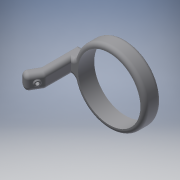
# Autodesk Inventor part: Layer1Gear
Saved by Autodesk Inventor 2019 (Build 230136000, 136)
## iProperties
Created: 2022-08-24
Part Number: Layer1Gear
Material: Generic
Document SubType Name: Modeling
Designer: zreik
Density: 1 g/cm^3
Appearance: Default
Author: zreik
Autodesk Inventor part; units mm, degrees
note: some values were not read from the file. Chosen so that the rebuilt part matches the saved one: sketch regions of "Extrusion1"; arc direction of "Extrusion1".
ref_plane "YZ Plane" through (0, 0, 0) normal (1, 0, 0) x (0, 1, 0)
ref_plane "XZ Plane" through (0, 0, 0) normal (0, 1, 0) x (-1, 0, 0)
ref_plane "XY Plane" through (0, 0, 0) normal (0, 0, 1) x (1, 0, 0)
sketch "Sketch1" plane through (0, 0, 0) normal (0, 0, 1) x (1, 0, 0)
  circle A0 centre (0, 0) radius 32.75
  circle A1 centre (0, 0) radius 37.75
  line L0 (-31.879657, 7.5) -> (-40, 7.5)
  line L1 (-40, 7.5) -> (-40, -7.5)
  line L2 (-40, -7.5) -> (-31.879657, -7.5)
  dimension "d0" = 65.5
  dimension "d1" = 75.5
  dimension "d4" = 15
  dimension "d5" = 40
  dimension "d6" = 7.5
  constraints: 6 end point, 2 centre point, 2 coincident, 2 perpendicular, 2 point on circle, 1 horizontal
  measures "d0" diameter of A0
  measures "d1" diameter of A1
  measures "d4" distance between parallel lines of L0 L2
  measures "d5" distance from line of point (0, 0) L1
  measures "d6" distance from line of point (0, 0) L0
extrude "Extrusion1" add sketch "Sketch1" along normal blind 17 contours A0 L0 A1 L2 | A0 L2 A1 L0 | A1 L2 L1 L0
chamfer "Chamfer1" distance 2 angle 45 2 edges at (-36.9975, 7.5, 8.5) (-36.9975, -7.5, 8.5)
fillet "Fillet1" radius 2 4 edges at (-38.9975, 7.5, 8.5) (-36.5483, 9.4489, 8.5) (-36.5483, -9.4489, 8.5) (-38.9975, -7.5, 8.5)
sketch "Sketch2" plane through (0, 0, 0) normal (0, 0, -1) x (-1, 0, 0)
  line L0 (40, 7.5) -> (40, -7.5)
  line L1 (40, -7.5) -> (50, -7.5)
  line L2 (50, -7.5) -> (50, 7.5)
  line L3 (50, 7.5) -> (40, 7.5)
  line L4 (40, 7.5) -> (40, -7.5)
  line L5 (39.696118, 7.5) -> (40, 7.5)
  point P0 (0, 0)
  point P1 (36.401408, 10)
  dimension "d11" = 10
  dimension "d12" = 0
  constraints: 8 end point, 2 parallel, 1 horizontal, 1 perpendicular, 1 other
  measures "d11" distance of L2.end L3.end
  measures "d12" vertical extent of L3
extrude "Extrusion2" add sketch "Sketch2" against normal blind 59
chamfer_without_effect "Chamfer2"
sketch "Sketch4" plane through (-41.339746, -7.5, 59) normal (-0.5, 0, 0.8660254) x (0.8660254, 0, 0.5)
  line L0 (0, 0) -> (-10, 0)
  line L1 (-10, 15) -> (0, 15)
  line L2 (-19.839746, 0) -> (1.160254, 0)
  line L3 (-37, 15) -> (-10, 15)
  line L4 (1.160254, 0) -> (-10, 0)
  line L5 (-10, 0) -> (-10, 15)
  line L6 (-10, 15) -> (1.160254, 15)
  line L7 (1.160254, 15) -> (1.160254, 0)
  point P0 (6.30127, 7.5)
  constraints: 12 end point, 3 parallel, 2 horizontal, 1 perpendicular
extrude "Extrusion4" add sketch "Sketch4" along normal blind 15
extrude "Extrusion5" add sketch "Sketch4" against normal up to next
fillet "Fillet3" radius 4 31 edges at (-40, 0, 59) (-40, 7.5, 38) (-36.6415, 9.5, 17) (37.75, 0, 17) (-36.6415, -9.5, 17) (-37.7576, -8.4867, 17) (-39.0366, -7.6119, 17) (-39.8481, -7.5, 17) (-39.0366, 7.6119, 17) (-39.8481, 7.5, 17) (-37.7576, 8.4867, 17) (-40, -7.5, 38) (-39.0366, -7.6119, 0) (-37.7576, -8.4867, 0) (-36.6415, -9.5, 0) (37.75, 0, 0) (-36.6415, 9.5, 0) (-37.7576, 8.4867, 0) (-39.0366, 7.6119, 0) (-44.8481, 7.5, 0) (-44.8481, -7.5, 0) (-50, -7.5, 27) (-50, 7.5, 27) (-53.75, -7.5, 60.4952) (-43.9175, -7.5, 65.7853) (-43.9175, 7.5, 65.7853) (-53.75, 7.5, 60.4952) (-52.6675, -7.5, 69.7804) (-52.6675, 7.5, 69.7804) (-47.8349, 0, 72.5705) (-57.5, 0, 66.9904)
sketch "Sketch5" plane through (-45.834936, -3.5, 69.106406) normal (0.8660254, 0, 0.5) x (0.5, 0, -0.8660254)
  circle A0 centre (5.299038, 3.5) radius 1.75
  circle A1 centre (5.299038, 3.5) radius 3.5
  line L0 (10.598076, 11) -> (0, 11)
  line L1 (0, -4) -> (10.598076, -4)
  line L2 (10.598076, 7) -> (10.598076, 0)
  line L3 (0, 0) -> (0, 7)
  point P0 (82.765372, 3.5)
  dimension "d30" = 7.5
  dimension "d31" = 7.5
  dimension "d32" = 5.29904
  dimension "d33" = 5.29904
  dimension "d34" = 3.5
  dimension "d35" = 7
  constraints: 2 centre point, 1 coincident
  measures "d30" distance from line of L0 A0.centre
  measures "d31" distance from line of A0.centre L1
  measures "d32" distance from line of L2 A0.centre
  measures "d33" distance from line of L3 A0.centre
  measures "d34" diameter of A0
  measures "d35" diameter of A1
extrude "Extrusion6" cut sketch "Sketch5" against normal blind 20 contours A0
extrude "Extrusion7" add sketch "Sketch5" along normal blind 1
chamfer "Chamfer3" distance 1 angle 45 1 edges at (-44.0694, 0, 68.0484)
equation "\"d6\" = 0.5 * d4"
equation "\"d30\" = d31"
equation "\"d32\" = d33"
body "Solid1"
